Autodesk Inventor part; units mm, degrees
(part 9 of 12)
  line L7174 (-19.2358, 25.9762) -> (-19.2358, 24.9762)
  line L7175 (-19.8581, 24.9762) -> (-20.8581, 24.9762)
  line L7176 (-20.8581, 24.9762) -> (-20.8581, 25.9762)
  line L7177 (-20.8581, 25.9762) -> (-19.8581, 25.9762)
  line L7178 (-19.8581, 25.9762) -> (-19.8581, 24.9762)
  line L7179 (-20.4804, 24.9762) -> (-21.4804, 24.9762)
  line L7180 (-21.4804, 24.9762) -> (-21.4804, 25.9762)
  line L7181 (-21.4804, 25.9762) -> (-20.4804, 25.9762)
  line L7182 (-20.4804, 25.9762) -> (-20.4804, 24.9762)
  line L7183 (-21.4837, 24.9762) -> (-22.4837, 24.9762)
  line L7184 (-22.4837, 24.9762) -> (-22.4837, 25.9762)
  line L7185 (-22.4837, 25.9762) -> (-21.4837, 25.9762)
  line L7186 (-21.4837, 25.9762) -> (-21.4837, 24.9762)
  line L7187 (-12.9239, 25.0016) -> (-13.9239, 25.0016)
  line L7188 (-13.9239, 25.0016) -> (-13.9239, 26.0016)
  line L7189 (-13.9239, 26.0016) -> (-12.9239, 26.0016)
  line L7190 (-12.9239, 26.0016) -> (-12.9239, 25.0016)
  line L7191 (-13.6478, 25.0016) -> (-14.6478, 25.0016)
  line L7192 (-14.6478, 25.0016) -> (-14.6478, 26.0016)
  line L7193 (-14.6478, 26.0016) -> (-13.6478, 26.0016)
  line L7194 (-13.6478, 26.0016) -> (-13.6478, 25.0016)
  line L7195 (-14.5622, 25.0016) -> (-15.5622, 25.0016)
  line L7196 (-15.5622, 25.0016) -> (-15.5622, 26.0016)
  line L7197 (-15.5622, 26.0016) -> (-14.5622, 26.0016)
  line L7198 (-14.5622, 26.0016) -> (-14.5622, 25.0016)
  line L7199 (-15.8449, 25.0016) -> (-16.8449, 25.0016)
  line L7200 (-16.8449, 25.0016) -> (-16.8449, 26.0016)
  line L7201 (-16.8449, 26.0016) -> (-15.8449, 26.0016)
  line L7202 (-15.8449, 26.0016) -> (-15.8449, 25.0016)
  line L7203 (-16.8228, 25.0016) -> (-17.8228, 25.0016)
  line L7204 (-17.8228, 25.0016) -> (-17.8228, 26.0016)
  line L7205 (-17.8228, 26.0016) -> (-16.8228, 26.0016)
  line L7206 (-16.8228, 26.0016) -> (-16.8228, 25.0016)
  line L7207 (-17.4324, 25.0016) -> (-18.4324, 25.0016)
  line L7208 (-18.4324, 25.0016) -> (-18.4324, 26.0016)
  line L7209 (-18.4324, 26.0016) -> (-17.4324, 26.0016)
  line L7210 (-17.4324, 26.0016) -> (-17.4324, 25.0016)
  line L7211 (-17.9404, 25.0016) -> (-18.9404, 25.0016)
  line L7212 (-18.9404, 25.0016) -> (-18.9404, 26.0016)
  line L7213 (-18.9404, 26.0016) -> (-17.9404, 26.0016)
  line L7214 (-17.9404, 26.0016) -> (-17.9404, 25.0016)
  line L7215 (-18.677, 25.0016) -> (-19.677, 25.0016)
  line L7216 (-19.677, 25.0016) -> (-19.677, 26.0016)
  line L7217 (-19.677, 26.0016) -> (-18.677, 26.0016)
  line L7218 (-18.677, 26.0016) -> (-18.677, 25.0016)
  line L7219 (-19.2485, 25.0016) -> (-20.2485, 25.0016)
  line L7220 (-20.2485, 25.0016) -> (-20.2485, 26.0016)
  line L7221 (-20.2485, 26.0016) -> (-19.2485, 26.0016)
  line L7222 (-19.2485, 26.0016) -> (-19.2485, 25.0016)
  line L7223 (-19.8454, 25.0016) -> (-20.8454, 25.0016)
  line L7224 (-20.8454, 25.0016) -> (-20.8454, 26.0016)
  line L7225 (-20.8454, 26.0016) -> (-19.8454, 26.0016)
  line L7226 (-19.8454, 26.0016) -> (-19.8454, 25.0016)
  line L7227 (-20.4804, 25.0016) -> (-21.4804, 25.0016)
  line L7228 (-21.4804, 25.0016) -> (-21.4804, 26.0016)
  line L7229 (-21.4804, 26.0016) -> (-20.4804, 26.0016)
  line L7230 (-20.4804, 26.0016) -> (-20.4804, 25.0016)
  line L7231 (-21.4837, 25.0016) -> (-22.4837, 25.0016)
  line L7232 (-22.4837, 25.0016) -> (-22.4837, 26.0016)
  line L7233 (-22.4837, 26.0016) -> (-21.4837, 26.0016)
  line L7234 (-21.4837, 26.0016) -> (-21.4837, 25.0016)
  line L7235 (-12.9239, 25.027) -> (-13.9239, 25.027)
  line L7236 (-13.9239, 25.027) -> (-13.9239, 26.027)
  line L7237 (-13.9239, 26.027) -> (-12.9239, 26.027)
  line L7238 (-12.9239, 26.027) -> (-12.9239, 25.027)
  line L7239 (-13.6224, 25.027) -> (-14.6224, 25.027)
  line L7240 (-14.6224, 25.027) -> (-14.6224, 26.027)
  line L7241 (-14.6224, 26.027) -> (-13.6224, 26.027)
  line L7242 (-13.6224, 26.027) -> (-13.6224, 25.027)
  line L7243 (-14.5495, 25.027) -> (-15.5495, 25.027)
  line L7244 (-15.5495, 25.027) -> (-15.5495, 26.027)
  line L7245 (-15.5495, 26.027) -> (-14.5495, 26.027)
  line L7246 (-14.5495, 26.027) -> (-14.5495, 25.027)
  line L7247 (-15.5528, 25.027) -> (-16.5528, 25.027)
  line L7248 (-16.5528, 25.027) -> (-16.5528, 26.027)
  line L7249 (-16.5528, 26.027) -> (-15.5528, 26.027)
  line L7250 (-15.5528, 26.027) -> (-15.5528, 25.027)
  line L7251 (-16.1751, 25.027) -> (-17.1751, 25.027)
  line L7252 (-17.1751, 25.027) -> (-17.1751, 26.027)
  line L7253 (-17.1751, 26.027) -> (-16.1751, 26.027)
  line L7254 (-16.1751, 26.027) -> (-16.1751, 25.027)
  line L7255 (-16.7974, 25.027) -> (-17.7974, 25.027)
  line L7256 (-17.7974, 25.027) -> (-17.7974, 26.027)
  line L7257 (-17.7974, 26.027) -> (-16.7974, 26.027)
  line L7258 (-16.7974, 26.027) -> (-16.7974, 25.027)
  line L7259 (-17.4832, 25.027) -> (-18.4832, 25.027)
  line L7260 (-18.4832, 25.027) -> (-18.4832, 26.027)
  line L7261 (-18.4832, 26.027) -> (-17.4832, 26.027)
  line L7262 (-17.4832, 26.027) -> (-17.4832, 25.027)
  line L7263 (-17.9404, 25.027) -> (-18.9404, 25.027)
  line L7264 (-18.9404, 25.027) -> (-18.9404, 26.027)
  line L7265 (-18.9404, 26.027) -> (-17.9404, 26.027)
  line L7266 (-17.9404, 26.027) -> (-17.9404, 25.027)
  line L7267 (-18.677, 25.027) -> (-19.677, 25.027)
  line L7268 (-19.677, 25.027) -> (-19.677, 26.027)
  line L7269 (-19.677, 26.027) -> (-18.677, 26.027)
  line L7270 (-18.677, 26.027) -> (-18.677, 25.027)
  line L7271 (-19.2485, 25.027) -> (-20.2485, 25.027)
  line L7272 (-20.2485, 25.027) -> (-20.2485, 26.027)
  line L7273 (-20.2485, 26.027) -> (-19.2485, 26.027)
  line L7274 (-19.2485, 26.027) -> (-19.2485, 25.027)
  line L7275 (-19.8581, 25.027) -> (-20.8581, 25.027)
  line L7276 (-20.8581, 25.027) -> (-20.8581, 26.027)
  line L7277 (-20.8581, 26.027) -> (-19.8581, 26.027)
  line L7278 (-19.8581, 26.027) -> (-19.8581, 25.027)
  line L7279 (-20.4804, 25.027) -> (-21.4804, 25.027)
  line L7280 (-21.4804, 25.027) -> (-21.4804, 26.027)
  line L7281 (-21.4804, 26.027) -> (-20.4804, 26.027)
  line L7282 (-20.4804, 26.027) -> (-20.4804, 25.027)
  line L7283 (-21.4964, 25.027) -> (-22.4964, 25.027)
  line L7284 (-22.4964, 25.027) -> (-22.4964, 26.027)
  line L7285 (-22.4964, 26.027) -> (-21.4964, 26.027)
  line L7286 (-21.4964, 26.027) -> (-21.4964, 25.027)
  line L7287 (-12.9112, 25.0524) -> (-13.9112, 25.0524)
  line L7288 (-13.9112, 25.0524) -> (-13.9112, 26.0524)
  line L7289 (-13.9112, 26.0524) -> (-12.9112, 26.0524)
  line L7290 (-12.9112, 26.0524) -> (-12.9112, 25.0524)
  line L7291 (-13.597, 25.0524) -> (-14.597, 25.0524)
  line L7292 (-14.597, 25.0524) -> (-14.597, 26.0524)
  line L7293 (-14.597, 26.0524) -> (-13.597, 26.0524)
  line L7294 (-13.597, 26.0524) -> (-13.597, 25.0524)
  line L7295 (-14.5241, 25.0524) -> (-15.5241, 25.0524)
  line L7296 (-15.5241, 25.0524) -> (-15.5241, 26.0524)
  line L7297 (-15.5241, 26.0524) -> (-14.5241, 26.0524)
  line L7298 (-14.5241, 26.0524) -> (-14.5241, 25.0524)
  line L7299 (-15.5274, 25.0524) -> (-16.5274, 25.0524)
  line L7300 (-16.5274, 25.0524) -> (-16.5274, 26.0524)
  line L7301 (-16.5274, 26.0524) -> (-15.5274, 26.0524)
  line L7302 (-15.5274, 26.0524) -> (-15.5274, 25.0524)
  line L7303 (-16.2005, 25.0524) -> (-17.2005, 25.0524)
  line L7304 (-17.2005, 25.0524) -> (-17.2005, 26.0524)
  line L7305 (-17.2005, 26.0524) -> (-16.2005, 26.0524)
  line L7306 (-16.2005, 26.0524) -> (-16.2005, 25.0524)
  line L7307 (-16.772, 25.0524) -> (-17.772, 25.0524)
  line L7308 (-17.772, 25.0524) -> (-17.772, 26.0524)
  line L7309 (-17.772, 26.0524) -> (-16.772, 26.0524)
  line L7310 (-16.772, 26.0524) -> (-16.772, 25.0524)
  line L7311 (-17.9404, 25.0524) -> (-18.9404, 25.0524)
  line L7312 (-18.9404, 25.0524) -> (-18.9404, 26.0524)
  line L7313 (-18.9404, 26.0524) -> (-17.9404, 26.0524)
  line L7314 (-17.9404, 26.0524) -> (-17.9404, 25.0524)
  line L7315 (-18.677, 25.0524) -> (-19.677, 25.0524)
  line L7316 (-19.677, 25.0524) -> (-19.677, 26.0524)
  line L7317 (-19.677, 26.0524) -> (-18.677, 26.0524)
  line L7318 (-18.677, 26.0524) -> (-18.677, 25.0524)
  line L7319 (-19.2485, 25.0524) -> (-20.2485, 25.0524)
  line L7320 (-20.2485, 25.0524) -> (-20.2485, 26.0524)
  line L7321 (-20.2485, 26.0524) -> (-19.2485, 26.0524)
  line L7322 (-19.2485, 26.0524) -> (-19.2485, 25.0524)
  line L7323 (-19.8581, 25.0524) -> (-20.8581, 25.0524)
  line L7324 (-20.8581, 25.0524) -> (-20.8581, 26.0524)
  line L7325 (-20.8581, 26.0524) -> (-19.8581, 26.0524)
  line L7326 (-19.8581, 26.0524) -> (-19.8581, 25.0524)
  line L7327 (-20.4804, 25.0524) -> (-21.4804, 25.0524)
  line L7328 (-21.4804, 25.0524) -> (-21.4804, 26.0524)
  line L7329 (-21.4804, 26.0524) -> (-20.4804, 26.0524)
  line L7330 (-20.4804, 26.0524) -> (-20.4804, 25.0524)
  line L7331 (-21.4837, 25.0524) -> (-22.4837, 25.0524)
  line L7332 (-22.4837, 25.0524) -> (-22.4837, 26.0524)
  line L7333 (-22.4837, 26.0524) -> (-21.4837, 26.0524)
  line L7334 (-21.4837, 26.0524) -> (-21.4837, 25.0524)
  line L7335 (-12.9112, 25.0778) -> (-13.9112, 25.0778)
  line L7336 (-13.9112, 25.0778) -> (-13.9112, 26.0778)
  line L7337 (-13.9112, 26.0778) -> (-12.9112, 26.0778)
  line L7338 (-12.9112, 26.0778) -> (-12.9112, 25.0778)
  line L7339 (-13.5843, 25.0778) -> (-14.5843, 25.0778)
  line L7340 (-14.5843, 25.0778) -> (-14.5843, 26.0778)
  line L7341 (-14.5843, 26.0778) -> (-13.5843, 26.0778)
  line L7342 (-13.5843, 26.0778) -> (-13.5843, 25.0778)
  line L7343 (-14.5241, 25.0778) -> (-15.5241, 25.0778)
  line L7344 (-15.5241, 25.0778) -> (-15.5241, 26.0778)
  line L7345 (-15.5241, 26.0778) -> (-14.5241, 26.0778)
  line L7346 (-14.5241, 26.0778) -> (-14.5241, 25.0778)
  line L7347 (-15.5147, 25.0778) -> (-16.5147, 25.0778)
  line L7348 (-16.5147, 25.0778) -> (-16.5147, 26.0778)
  line L7349 (-16.5147, 26.0778) -> (-15.5147, 26.0778)
  line L7350 (-15.5147, 26.0778) -> (-15.5147, 25.0778)
  line L7351 (-16.2005, 25.0778) -> (-17.2005, 25.0778)
  line L7352 (-17.2005, 25.0778) -> (-17.2005, 26.0778)
  line L7353 (-17.2005, 26.0778) -> (-16.2005, 26.0778)
  line L7354 (-16.2005, 26.0778) -> (-16.2005, 25.0778)
  line L7355 (-16.7466, 25.0778) -> (-17.7466, 25.0778)
  line L7356 (-17.7466, 25.0778) -> (-17.7466, 26.0778)
  line L7357 (-17.7466, 26.0778) -> (-16.7466, 26.0778)
  line L7358 (-16.7466, 26.0778) -> (-16.7466, 25.0778)
  line L7359 (-17.9404, 25.0778) -> (-18.9404, 25.0778)
  line L7360 (-18.9404, 25.0778) -> (-18.9404, 26.0778)
  line L7361 (-18.9404, 26.0778) -> (-17.9404, 26.0778)
  line L7362 (-17.9404, 26.0778) -> (-17.9404, 25.0778)
  line L7363 (-18.677, 25.0778) -> (-19.677, 25.0778)
  line L7364 (-19.677, 25.0778) -> (-19.677, 26.0778)
  line L7365 (-19.677, 26.0778) -> (-18.677, 26.0778)
  line L7366 (-18.677, 26.0778) -> (-18.677, 25.0778)
  line L7367 (-19.2485, 25.0778) -> (-20.2485, 25.0778)
  line L7368 (-20.2485, 25.0778) -> (-20.2485, 26.0778)
  line L7369 (-20.2485, 26.0778) -> (-19.2485, 26.0778)
  line L7370 (-19.2485, 26.0778) -> (-19.2485, 25.0778)
  line L7371 (-19.8581, 25.0778) -> (-20.8581, 25.0778)
  line L7372 (-20.8581, 25.0778) -> (-20.8581, 26.0778)
  line L7373 (-20.8581, 26.0778) -> (-19.8581, 26.0778)
  line L7374 (-19.8581, 26.0778) -> (-19.8581, 25.0778)
  line L7375 (-20.4804, 25.0778) -> (-21.4804, 25.0778)
  line L7376 (-21.4804, 25.0778) -> (-21.4804, 26.0778)
  line L7377 (-21.4804, 26.0778) -> (-20.4804, 26.0778)
  line L7378 (-20.4804, 26.0778) -> (-20.4804, 25.0778)
  line L7379 (-21.4964, 25.0778) -> (-22.4964, 25.0778)
  line L7380 (-22.4964, 25.0778) -> (-22.4964, 26.0778)
  line L7381 (-22.4964, 26.0778) -> (-21.4964, 26.0778)
  line L7382 (-21.4964, 26.0778) -> (-21.4964, 25.0778)
  line L7383 (-12.8985, 25.1032) -> (-13.8985, 25.1032)
  line L7384 (-13.8985, 25.1032) -> (-13.8985, 26.1032)
  line L7385 (-13.8985, 26.1032) -> (-12.8985, 26.1032)
  line L7386 (-12.8985, 26.1032) -> (-12.8985, 25.1032)
  line L7387 (-13.5589, 25.1032) -> (-14.5589, 25.1032)
  line L7388 (-14.5589, 25.1032) -> (-14.5589, 26.1032)
  line L7389 (-14.5589, 26.1032) -> (-13.5589, 26.1032)
  line L7390 (-13.5589, 26.1032) -> (-13.5589, 25.1032)
  line L7391 (-14.4987, 25.1032) -> (-15.4987, 25.1032)
  line L7392 (-15.4987, 25.1032) -> (-15.4987, 26.1032)
  line L7393 (-15.4987, 26.1032) -> (-14.4987, 26.1032)
  line L7394 (-14.4987, 26.1032) -> (-14.4987, 25.1032)
  line L7395 (-15.5147, 25.1032) -> (-16.5147, 25.1032)
  line L7396 (-16.5147, 25.1032) -> (-16.5147, 26.1032)
  line L7397 (-16.5147, 26.1032) -> (-15.5147, 26.1032)
  line L7398 (-15.5147, 26.1032) -> (-15.5147, 25.1032)
  line L7399 (-16.2132, 25.1032) -> (-17.2132, 25.1032)
  line L7400 (-17.2132, 25.1032) -> (-17.2132, 26.1032)
  line L7401 (-17.2132, 26.1032) -> (-16.2132, 26.1032)
  line L7402 (-16.2132, 26.1032) -> (-16.2132, 25.1032)
  line L7403 (-16.7466, 25.1032) -> (-17.7466, 25.1032)
  line L7404 (-17.7466, 25.1032) -> (-17.7466, 26.1032)
  line L7405 (-17.7466, 26.1032) -> (-16.7466, 26.1032)
  line L7406 (-16.7466, 26.1032) -> (-16.7466, 25.1032)
  line L7407 (-17.9404, 25.1032) -> (-18.9404, 25.1032)
  line L7408 (-18.9404, 25.1032) -> (-18.9404, 26.1032)
  line L7409 (-18.9404, 26.1032) -> (-17.9404, 26.1032)
  line L7410 (-17.9404, 26.1032) -> (-17.9404, 25.1032)
  line L7411 (-18.677, 25.1032) -> (-19.677, 25.1032)
  line L7412 (-19.677, 25.1032) -> (-19.677, 26.1032)
  line L7413 (-19.677, 26.1032) -> (-18.677, 26.1032)
  line L7414 (-18.677, 26.1032) -> (-18.677, 25.1032)
  line L7415 (-19.2485, 25.1032) -> (-20.2485, 25.1032)
  line L7416 (-20.2485, 25.1032) -> (-20.2485, 26.1032)
  line L7417 (-20.2485, 26.1032) -> (-19.2485, 26.1032)
  line L7418 (-19.2485, 26.1032) -> (-19.2485, 25.1032)
  line L7419 (-19.8581, 25.1032) -> (-20.8581, 25.1032)
  line L7420 (-20.8581, 25.1032) -> (-20.8581, 26.1032)
  line L7421 (-20.8581, 26.1032) -> (-19.8581, 26.1032)
  line L7422 (-19.8581, 26.1032) -> (-19.8581, 25.1032)
  line L7423 (-20.4804, 25.1032) -> (-21.4804, 25.1032)
  line L7424 (-21.4804, 25.1032) -> (-21.4804, 26.1032)
  line L7425 (-21.4804, 26.1032) -> (-20.4804, 26.1032)
  line L7426 (-20.4804, 26.1032) -> (-20.4804, 25.1032)
  line L7427 (-21.3059, 25.1032) -> (-22.3059, 25.1032)
  line L7428 (-22.3059, 25.1032) -> (-22.3059, 26.1032)
  line L7429 (-22.3059, 26.1032) -> (-21.3059, 26.1032)
  line L7430 (-21.3059, 26.1032) -> (-21.3059, 25.1032)
  line L7431 (-21.6869, 25.1032) -> (-22.6869, 25.1032)
  line L7432 (-22.6869, 25.1032) -> (-22.6869, 26.1032)
  line L7433 (-22.6869, 26.1032) -> (-21.6869, 26.1032)
  line L7434 (-21.6869, 26.1032) -> (-21.6869, 25.1032)
  line L7435 (-12.8985, 25.1286) -> (-13.8985, 25.1286)
  line L7436 (-13.8985, 25.1286) -> (-13.8985, 26.1286)
  line L7437 (-13.8985, 26.1286) -> (-12.8985, 26.1286)
  line L7438 (-12.8985, 26.1286) -> (-12.8985, 25.1286)
  line L7439 (-13.5335, 25.1286) -> (-14.5335, 25.1286)
  line L7440 (-14.5335, 25.1286) -> (-14.5335, 26.1286)
  line L7441 (-14.5335, 26.1286) -> (-13.5335, 26.1286)
  line L7442 (-13.5335, 26.1286) -> (-13.5335, 25.1286)
  line L7443 (-14.486, 25.1286) -> (-15.486, 25.1286)
  line L7444 (-15.486, 25.1286) -> (-15.486, 26.1286)
  line L7445 (-15.486, 26.1286) -> (-14.486, 26.1286)
  line L7446 (-14.486, 26.1286) -> (-14.486, 25.1286)
  line L7447 (-15.502, 25.1286) -> (-16.502, 25.1286)
  line L7448 (-16.502, 25.1286) -> (-16.502, 26.1286)
  line L7449 (-16.502, 26.1286) -> (-15.502, 26.1286)
  line L7450 (-15.502, 26.1286) -> (-15.502, 25.1286)
  line L7451 (-16.2386, 25.1286) -> (-17.2386, 25.1286)
  line L7452 (-17.2386, 25.1286) -> (-17.2386, 26.1286)
  line L7453 (-17.2386, 26.1286) -> (-16.2386, 26.1286)
  line L7454 (-16.2386, 26.1286) -> (-16.2386, 25.1286)
  line L7455 (-16.7466, 25.1286) -> (-17.7466, 25.1286)
  line L7456 (-17.7466, 25.1286) -> (-17.7466, 26.1286)
  line L7457 (-17.7466, 26.1286) -> (-16.7466, 26.1286)
  line L7458 (-16.7466, 26.1286) -> (-16.7466, 25.1286)
  line L7459 (-17.9404, 25.1286) -> (-18.9404, 25.1286)
  line L7460 (-18.9404, 25.1286) -> (-18.9404, 26.1286)
  line L7461 (-18.9404, 26.1286) -> (-17.9404, 26.1286)
  line L7462 (-17.9404, 26.1286) -> (-17.9404, 25.1286)
  line L7463 (-18.677, 25.1286) -> (-19.677, 25.1286)
  line L7464 (-19.677, 25.1286) -> (-19.677, 26.1286)
  line L7465 (-19.677, 26.1286) -> (-18.677, 26.1286)
  line L7466 (-18.677, 26.1286) -> (-18.677, 25.1286)
  line L7467 (-19.2485, 25.1286) -> (-20.2485, 25.1286)
  line L7468 (-20.2485, 25.1286) -> (-20.2485, 26.1286)
  line L7469 (-20.2485, 26.1286) -> (-19.2485, 26.1286)
  line L7470 (-19.2485, 26.1286) -> (-19.2485, 25.1286)
  line L7471 (-19.8581, 25.1286) -> (-20.8581, 25.1286)
  line L7472 (-20.8581, 25.1286) -> (-20.8581, 26.1286)
  line L7473 (-20.8581, 26.1286) -> (-19.8581, 26.1286)
  line L7474 (-19.8581, 26.1286) -> (-19.8581, 25.1286)
  line L7475 (-20.4804, 25.1286) -> (-21.4804, 25.1286)
  line L7476 (-21.4804, 25.1286) -> (-21.4804, 26.1286)
  line L7477 (-21.4804, 26.1286) -> (-20.4804, 26.1286)
  line L7478 (-20.4804, 26.1286) -> (-20.4804, 25.1286)
  line L7479 (-21.2932, 25.1286) -> (-22.2932, 25.1286)
  line L7480 (-22.2932, 25.1286) -> (-22.2932, 26.1286)
  line L7481 (-22.2932, 26.1286) -> (-21.2932, 26.1286)
  line L7482 (-21.2932, 26.1286) -> (-21.2932, 25.1286)
  line L7483 (-21.6996, 25.1286) -> (-22.6996, 25.1286)
  line L7484 (-22.6996, 25.1286) -> (-22.6996, 26.1286)
  line L7485 (-22.6996, 26.1286) -> (-21.6996, 26.1286)
  line L7486 (-21.6996, 26.1286) -> (-21.6996, 25.1286)
  line L7487 (-12.8858, 25.154) -> (-13.8858, 25.154)
  line L7488 (-13.8858, 25.154) -> (-13.8858, 26.154)
  line L7489 (-13.8858, 26.154) -> (-12.8858, 26.154)
  line L7490 (-12.8858, 26.154) -> (-12.8858, 25.154)
  line L7491 (-13.5208, 25.154) -> (-14.5208, 25.154)
  line L7492 (-14.5208, 25.154) -> (-14.5208, 26.154)
  line L7493 (-14.5208, 26.154) -> (-13.5208, 26.154)
  line L7494 (-13.5208, 26.154) -> (-13.5208, 25.154)
  line L7495 (-14.4606, 25.154) -> (-15.4606, 25.154)
  line L7496 (-15.4606, 25.154) -> (-15.4606, 26.154)
  line L7497 (-15.4606, 26.154) -> (-14.4606, 26.154)
  line L7498 (-14.4606, 26.154) -> (-14.4606, 25.154)
  line L7499 (-15.502, 25.154) -> (-16.502, 25.154)
  line L7500 (-16.502, 25.154) -> (-16.502, 26.154)
  line L7501 (-16.502, 26.154) -> (-15.502, 26.154)
  line L7502 (-15.502, 26.154) -> (-15.502, 25.154)
  line L7503 (-16.2386, 25.154) -> (-17.2386, 25.154)
  line L7504 (-17.2386, 25.154) -> (-17.2386, 26.154)
  line L7505 (-17.2386, 26.154) -> (-16.2386, 26.154)
  line L7506 (-16.2386, 26.154) -> (-16.2386, 25.154)
  line L7507 (-16.7339, 25.154) -> (-17.7339, 25.154)
  line L7508 (-17.7339, 25.154) -> (-17.7339, 26.154)
  line L7509 (-17.7339, 26.154) -> (-16.7339, 26.154)
  line L7510 (-16.7339, 26.154) -> (-16.7339, 25.154)
  line L7511 (-17.9531, 25.154) -> (-18.9531, 25.154)
  line L7512 (-18.9531, 25.154) -> (-18.9531, 26.154)
  line L7513 (-18.9531, 26.154) -> (-17.9531, 26.154)
  line L7514 (-17.9531, 26.154) -> (-17.9531, 25.154)
  line L7515 (-18.677, 25.154) -> (-19.677, 25.154)
  line L7516 (-19.677, 25.154) -> (-19.677, 26.154)
  line L7517 (-19.677, 26.154) -> (-18.677, 26.154)
  line L7518 (-18.677, 26.154) -> (-18.677, 25.154)
  line L7519 (-19.2485, 25.154) -> (-20.2485, 25.154)
  line L7520 (-20.2485, 25.154) -> (-20.2485, 26.154)
  line L7521 (-20.2485, 26.154) -> (-19.2485, 26.154)
  line L7522 (-19.2485, 26.154) -> (-19.2485, 25.154)
  line L7523 (-19.8581, 25.154) -> (-20.8581, 25.154)
  line L7524 (-20.8581, 25.154) -> (-20.8581, 26.154)
  line L7525 (-20.8581, 26.154) -> (-19.8581, 26.154)
  line L7526 (-19.8581, 26.154) -> (-19.8581, 25.154)
  line L7527 (-20.4804, 25.154) -> (-21.4804, 25.154)
  line L7528 (-21.4804, 25.154) -> (-21.4804, 26.154)
  line L7529 (-21.4804, 26.154) -> (-20.4804, 26.154)
  line L7530 (-20.4804, 26.154) -> (-20.4804, 25.154)
  line L7531 (-21.2932, 25.154) -> (-22.2932, 25.154)
  line L7532 (-22.2932, 25.154) -> (-22.2932, 26.154)
  line L7533 (-22.2932, 26.154) -> (-21.2932, 26.154)
  line L7534 (-21.2932, 26.154) -> (-21.2932, 25.154)
  line L7535 (-21.7123, 25.154) -> (-22.7123, 25.154)
  line L7536 (-22.7123, 25.154) -> (-22.7123, 26.154)
  line L7537 (-22.7123, 26.154) -> (-21.7123, 26.154)
  line L7538 (-21.7123, 26.154) -> (-21.7123, 25.154)
  line L7539 (-12.8858, 25.1794) -> (-13.8858, 25.1794)
  line L7540 (-13.8858, 25.1794) -> (-13.8858, 26.1794)
  line L7541 (-13.8858, 26.1794) -> (-12.8858, 26.1794)
  line L7542 (-12.8858, 26.1794) -> (-12.8858, 25.1794)
  line L7543 (-13.4954, 25.1794) -> (-14.4954, 25.1794)
  line L7544 (-14.4954, 25.1794) -> (-14.4954, 26.1794)
  line L7545 (-14.4954, 26.1794) -> (-13.4954, 26.1794)
  line L7546 (-13.4954, 26.1794) -> (-13.4954, 25.1794)
  line L7547 (-14.4733, 25.1794) -> (-15.4733, 25.1794)
  line L7548 (-15.4733, 25.1794) -> (-15.4733, 26.1794)
  line L7549 (-15.4733, 26.1794) -> (-14.4733, 26.1794)
  line L7550 (-14.4733, 26.1794) -> (-14.4733, 25.1794)
  line L7551 (-15.502, 25.1794) -> (-16.502, 25.1794)
  line L7552 (-16.502, 25.1794) -> (-16.502, 26.1794)
  line L7553 (-16.502, 26.1794) -> (-15.502, 26.1794)
  line L7554 (-15.502, 26.1794) -> (-15.502, 25.1794)
  line L7555 (-16.2386, 25.1794) -> (-17.2386, 25.1794)
  line L7556 (-17.2386, 25.1794) -> (-17.2386, 26.1794)
  line L7557 (-17.2386, 26.1794) -> (-16.2386, 26.1794)
  line L7558 (-16.2386, 26.1794) -> (-16.2386, 25.1794)
  line L7559 (-16.7339, 25.1794) -> (-17.7339, 25.1794)
  line L7560 (-17.7339, 25.1794) -> (-17.7339, 26.1794)
  line L7561 (-17.7339, 26.1794) -> (-16.7339, 26.1794)
  line L7562 (-16.7339, 26.1794) -> (-16.7339, 25.1794)
  line L7563 (-17.9531, 25.1794) -> (-18.9531, 25.1794)
  line L7564 (-18.9531, 25.1794) -> (-18.9531, 26.1794)
  line L7565 (-18.9531, 26.1794) -> (-17.9531, 26.1794)
  line L7566 (-17.9531, 26.1794) -> (-17.9531, 25.1794)
  line L7567 (-18.677, 25.1794) -> (-19.677, 25.1794)
  line L7568 (-19.677, 25.1794) -> (-19.677, 26.1794)
  line L7569 (-19.677, 26.1794) -> (-18.677, 26.1794)
  line L7570 (-18.677, 26.1794) -> (-18.677, 25.1794)
  line L7571 (-19.2485, 25.1794) -> (-20.2485, 25.1794)
  line L7572 (-20.2485, 25.1794) -> (-20.2485, 26.1794)
  line L7573 (-20.2485, 26.1794) -> (-19.2485, 26.1794)
  line L7574 (-19.2485, 26.1794) -> (-19.2485, 25.1794)
  line L7575 (-19.8708, 25.1794) -> (-20.8708, 25.1794)
  line L7576 (-20.8708, 25.1794) -> (-20.8708, 26.1794)
  line L7577 (-20.8708, 26.1794) -> (-19.8708, 26.1794)
  line L7578 (-19.8708, 26.1794) -> (-19.8708, 25.1794)
  line L7579 (-20.4804, 25.1794) -> (-21.4804, 25.1794)
  line L7580 (-21.4804, 25.1794) -> (-21.4804, 26.1794)
  line L7581 (-21.4804, 26.1794) -> (-20.4804, 26.1794)
  line L7582 (-20.4804, 26.1794) -> (-20.4804, 25.1794)
  line L7583 (-21.2805, 25.1794) -> (-22.2805, 25.1794)
  line L7584 (-22.2805, 25.1794) -> (-22.2805, 26.1794)
  line L7585 (-22.2805, 26.1794) -> (-21.2805, 26.1794)
  line L7586 (-21.2805, 26.1794) -> (-21.2805, 25.1794)
  line L7587 (-21.725, 25.1794) -> (-22.725, 25.1794)
  line L7588 (-22.725, 25.1794) -> (-22.725, 26.1794)
  line L7589 (-22.725, 26.1794) -> (-21.725, 26.1794)
  line L7590 (-21.725, 26.1794) -> (-21.725, 25.1794)
  line L7591 (-12.8731, 25.2048) -> (-13.8731, 25.2048)
  line L7592 (-13.8731, 25.2048) -> (-13.8731, 26.2048)
  line L7593 (-13.8731, 26.2048) -> (-12.8731, 26.2048)
  line L7594 (-12.8731, 26.2048) -> (-12.8731, 25.2048)
  line L7595 (-13.47, 25.2048) -> (-14.47, 25.2048)
  line L7596 (-14.47, 25.2048) -> (-14.47, 26.2048)
  line L7597 (-14.47, 26.2048) -> (-13.47, 26.2048)
  line L7598 (-13.47, 26.2048) -> (-13.47, 25.2048)
  line L7599 (-14.4987, 25.2048) -> (-15.4987, 25.2048)
  line L7600 (-15.4987, 25.2048) -> (-15.4987, 26.2048)
  line L7601 (-15.4987, 26.2048) -> (-14.4987, 26.2048)
  line L7602 (-14.4987, 26.2048) -> (-14.4987, 25.2048)
  line L7603 (-15.502, 25.2048) -> (-16.502, 25.2048)
  line L7604 (-16.502, 25.2048) -> (-16.502, 26.2048)
  line L7605 (-16.502, 26.2048) -> (-15.502, 26.2048)
  line L7606 (-15.502, 26.2048) -> (-15.502, 25.2048)
  line L7607 (-16.2386, 25.2048) -> (-17.2386, 25.2048)
  line L7608 (-17.2386, 25.2048) -> (-17.2386, 26.2048)
  line L7609 (-17.2386, 26.2048) -> (-16.2386, 26.2048)
  line L7610 (-16.2386, 26.2048) -> (-16.2386, 25.2048)
  line L7611 (-16.7339, 25.2048) -> (-17.7339, 25.2048)
  line L7612 (-17.7339, 25.2048) -> (-17.7339, 26.2048)
  line L7613 (-17.7339, 26.2048) -> (-16.7339, 26.2048)
  line L7614 (-16.7339, 26.2048) -> (-16.7339, 25.2048)
  line L7615 (-17.9531, 25.2048) -> (-18.9531, 25.2048)
  line L7616 (-18.9531, 25.2048) -> (-18.9531, 26.2048)
  line L7617 (-18.9531, 26.2048) -> (-17.9531, 26.2048)
  line L7618 (-17.9531, 26.2048) -> (-17.9531, 25.2048)
  line L7619 (-18.677, 25.2048) -> (-19.677, 25.2048)
  line L7620 (-19.677, 25.2048) -> (-19.677, 26.2048)
  line L7621 (-19.677, 26.2048) -> (-18.677, 26.2048)
  line L7622 (-18.677, 26.2048) -> (-18.677, 25.2048)
  line L7623 (-19.2612, 25.2048) -> (-20.2612, 25.2048)
  line L7624 (-20.2612, 25.2048) -> (-20.2612, 26.2048)
  line L7625 (-20.2612, 26.2048) -> (-19.2612, 26.2048)
  line L7626 (-19.2612, 26.2048) -> (-19.2612, 25.2048)
  line L7627 (-19.8708, 25.2048) -> (-20.8708, 25.2048)
  line L7628 (-20.8708, 25.2048) -> (-20.8708, 26.2048)
  line L7629 (-20.8708, 26.2048) -> (-19.8708, 26.2048)
  line L7630 (-19.8708, 26.2048) -> (-19.8708, 25.2048)
  line L7631 (-20.4804, 25.2048) -> (-21.4804, 25.2048)
  line L7632 (-21.4804, 25.2048) -> (-21.4804, 26.2048)
  line L7633 (-21.4804, 26.2048) -> (-20.4804, 26.2048)
  line L7634 (-20.4804, 26.2048) -> (-20.4804, 25.2048)
  line L7635 (-21.2678, 25.2048) -> (-22.2678, 25.2048)
  line L7636 (-22.2678, 25.2048) -> (-22.2678, 26.2048)
  line L7637 (-22.2678, 26.2048) -> (-21.2678, 26.2048)
  line L7638 (-21.2678, 26.2048) -> (-21.2678, 25.2048)
  line L7639 (-21.725, 25.2048) -> (-22.725, 25.2048)
  line L7640 (-22.725, 25.2048) -> (-22.725, 26.2048)
  line L7641 (-22.725, 26.2048) -> (-21.725, 26.2048)
  line L7642 (-21.725, 26.2048) -> (-21.725, 25.2048)
  line L7643 (-12.8731, 25.2302) -> (-13.8731, 25.2302)
  line L7644 (-13.8731, 25.2302) -> (-13.8731, 26.2302)
  line L7645 (-13.8731, 26.2302) -> (-12.8731, 26.2302)
  line L7646 (-12.8731, 26.2302) -> (-12.8731, 25.2302)
  line L7647 (-13.9319, 25.7175) -> (-13.9573, 25.7175)
  line L7648 (-13.9573, 25.7175) -> (-13.9573, 25.7429)
  line L7649 (-13.9573, 25.7429) -> (-13.9319, 25.7429)
  line L7650 (-13.9319, 25.7429) -> (-13.9319, 25.7175)
  line L7651 (-14.5241, 25.2302) -> (-15.5241, 25.2302)
  line L7652 (-15.5241, 25.2302) -> (-15.5241, 26.2302)
  line L7653 (-15.5241, 26.2302) -> (-14.5241, 26.2302)
  line L7654 (-14.5241, 26.2302) -> (-14.5241, 25.2302)
  line L7655 (-15.4893, 25.2302) -> (-16.4893, 25.2302)
  line L7656 (-16.4893, 25.2302) -> (-16.4893, 26.2302)
  line L7657 (-16.4893, 26.2302) -> (-15.4893, 26.2302)
  line L7658 (-15.4893, 26.2302) -> (-15.4893, 25.2302)
  line L7659 (-16.2386, 25.2302) -> (-17.2386, 25.2302)
  line L7660 (-17.2386, 25.2302) -> (-17.2386, 26.2302)
  line L7661 (-17.2386, 26.2302) -> (-16.2386, 26.2302)
  line L7662 (-16.2386, 26.2302) -> (-16.2386, 25.2302)
  line L7663 (-17.0768, 25.2302) -> (-18.0768, 25.2302)
  line L7664 (-18.0768, 25.2302) -> (-18.0768, 26.2302)
  line L7665 (-18.0768, 26.2302) -> (-17.0768, 26.2302)
  line L7666 (-17.0768, 26.2302) -> (-17.0768, 25.2302)
  line L7667 (-17.9658, 25.2302) -> (-18.9658, 25.2302)
  line L7668 (-18.9658, 25.2302) -> (-18.9658, 26.2302)
  line L7669 (-18.9658, 26.2302) -> (-17.9658, 26.2302)
  line L7670 (-17.9658, 26.2302) -> (-17.9658, 25.2302)
  line L7671 (-18.6897, 25.2302) -> (-19.6897, 25.2302)
  line L7672 (-19.6897, 25.2302) -> (-19.6897, 26.2302)
  line L7673 (-19.6897, 26.2302) -> (-18.6897, 26.2302)
  line L7674 (-18.6897, 26.2302) -> (-18.6897, 25.2302)
  line L7675 (-19.2612, 25.2302) -> (-20.2612, 25.2302)
  line L7676 (-20.2612, 25.2302) -> (-20.2612, 26.2302)
  line L7677 (-20.2612, 26.2302) -> (-19.2612, 26.2302)
  line L7678 (-19.2612, 26.2302) -> (-19.2612, 25.2302)
  line L7679 (-19.8581, 25.2302) -> (-20.8581, 25.2302)
  line L7680 (-20.8581, 25.2302) -> (-20.8581, 26.2302)
  line L7681 (-20.8581, 26.2302) -> (-19.8581, 26.2302)
  line L7682 (-19.8581, 26.2302) -> (-19.8581, 25.2302)
  line L7683 (-20.4804, 25.2302) -> (-21.4804, 25.2302)
  line L7684 (-21.4804, 25.2302) -> (-21.4804, 26.2302)
  line L7685 (-21.4804, 26.2302) -> (-20.4804, 26.2302)
  line L7686 (-20.4804, 26.2302) -> (-20.4804, 25.2302)
  line L7687 (-21.2678, 25.2302) -> (-22.2678, 25.2302)
  line L7688 (-22.2678, 25.2302) -> (-22.2678, 26.2302)
  line L7689 (-22.2678, 26.2302) -> (-21.2678, 26.2302)
  line L7690 (-21.2678, 26.2302) -> (-21.2678, 25.2302)
  line L7691 (-21.7504, 25.2302) -> (-22.7504, 25.2302)
  line L7692 (-22.7504, 25.2302) -> (-22.7504, 26.2302)
  line L7693 (-22.7504, 26.2302) -> (-21.7504, 26.2302)
  line L7694 (-21.7504, 26.2302) -> (-21.7504, 25.2302)
  line L7695 (-12.8731, 25.2556) -> (-13.8731, 25.2556)
  line L7696 (-13.8731, 25.2556) -> (-13.8731, 26.2556)
  line L7697 (-13.8731, 26.2556) -> (-12.8731, 26.2556)
  line L7698 (-12.8731, 26.2556) -> (-12.8731, 25.2556)
  line L7699 (-14.5495, 25.2556) -> (-15.5495, 25.2556)
  line L7700 (-15.5495, 25.2556) -> (-15.5495, 26.2556)
  line L7701 (-15.5495, 26.2556) -> (-14.5495, 26.2556)
  line L7702 (-14.5495, 26.2556) -> (-14.5495, 25.2556)
  line L7703 (-15.4893, 25.2556) -> (-16.4893, 25.2556)
  line L7704 (-16.4893, 25.2556) -> (-16.4893, 26.2556)
  line L7705 (-16.4893, 26.2556) -> (-15.4893, 26.2556)
  line L7706 (-15.4893, 26.2556) -> (-15.4893, 25.2556)
  line L7707 (-16.2386, 25.2556) -> (-17.2386, 25.2556)
  line L7708 (-17.2386, 25.2556) -> (-17.2386, 26.2556)
  line L7709 (-17.2386, 26.2556) -> (-16.2386, 26.2556)
  line L7710 (-16.2386, 26.2556) -> (-16.2386, 25.2556)
  line L7711 (-17.0768, 25.2556) -> (-18.0768, 25.2556)
  line L7712 (-18.0768, 25.2556) -> (-18.0768, 26.2556)
  line L7713 (-18.0768, 26.2556) -> (-17.0768, 26.2556)
  line L7714 (-17.0768, 26.2556) -> (-17.0768, 25.2556)
  line L7715 (-17.9658, 25.2556) -> (-18.9658, 25.2556)
  line L7716 (-18.9658, 25.2556) -> (-18.9658, 26.2556)
  line L7717 (-18.9658, 26.2556) -> (-17.9658, 26.2556)
  line L7718 (-17.9658, 26.2556) -> (-17.9658, 25.2556)
  line L7719 (-18.6897, 25.2556) -> (-19.6897, 25.2556)
  line L7720 (-19.6897, 25.2556) -> (-19.6897, 26.2556)
  line L7721 (-19.6897, 26.2556) -> (-18.6897, 26.2556)
  line L7722 (-18.6897, 26.2556) -> (-18.6897, 25.2556)
  line L7723 (-19.2612, 25.2556) -> (-20.2612, 25.2556)
  line L7724 (-20.2612, 25.2556) -> (-20.2612, 26.2556)
  line L7725 (-20.2612, 26.2556) -> (-19.2612, 26.2556)
  line L7726 (-19.2612, 26.2556) -> (-19.2612, 25.2556)
  line L7727 (-19.8708, 25.2556) -> (-20.8708, 25.2556)
  line L7728 (-20.8708, 25.2556) -> (-20.8708, 26.2556)
  line L7729 (-20.8708, 26.2556) -> (-19.8708, 26.2556)
  line L7730 (-19.8708, 26.2556) -> (-19.8708, 25.2556)
  line L7731 (-20.4804, 25.2556) -> (-21.4804, 25.2556)
  line L7732 (-21.4804, 25.2556) -> (-21.4804, 26.2556)
  line L7733 (-21.4804, 26.2556) -> (-20.4804, 26.2556)
  line L7734 (-20.4804, 26.2556) -> (-20.4804, 25.2556)
  line L7735 (-21.2678, 25.2556) -> (-22.2678, 25.2556)
  line L7736 (-22.2678, 25.2556) -> (-22.2678, 26.2556)
  line L7737 (-22.2678, 26.2556) -> (-21.2678, 26.2556)
  line L7738 (-21.2678, 26.2556) -> (-21.2678, 25.2556)
  line L7739 (-21.7504, 25.2556) -> (-22.7504, 25.2556)
  line L7740 (-22.7504, 25.2556) -> (-22.7504, 26.2556)
  line L7741 (-22.7504, 26.2556) -> (-21.7504, 26.2556)
  line L7742 (-21.7504, 26.2556) -> (-21.7504, 25.2556)
  line L7743 (-12.8731, 25.281) -> (-13.8731, 25.281)
  line L7744 (-13.8731, 25.281) -> (-13.8731, 26.281)
  line L7745 (-13.8731, 26.281) -> (-12.8731, 26.281)
  line L7746 (-12.8731, 26.281) -> (-12.8731, 25.281)
  line L7747 (-14.5749, 25.281) -> (-15.5749, 25.281)
  line L7748 (-15.5749, 25.281) -> (-15.5749, 26.281)
  line L7749 (-15.5749, 26.281) -> (-14.5749, 26.281)
  line L7750 (-14.5749, 26.281) -> (-14.5749, 25.281)
  line L7751 (-15.4893, 25.281) -> (-16.4893, 25.281)
  line L7752 (-16.4893, 25.281) -> (-16.4893, 26.281)
  line L7753 (-16.4893, 26.281) -> (-15.4893, 26.281)
  line L7754 (-15.4893, 26.281) -> (-15.4893, 25.281)
  line L7755 (-16.2386, 25.281) -> (-17.2386, 25.281)
  line L7756 (-17.2386, 25.281) -> (-17.2386, 26.281)
  line L7757 (-17.2386, 26.281) -> (-16.2386, 26.281)
  line L7758 (-16.2386, 26.281) -> (-16.2386, 25.281)
  line L7759 (-17.0768, 25.281) -> (-18.0768, 25.281)
  line L7760 (-18.0768, 25.281) -> (-18.0768, 26.281)
  line L7761 (-18.0768, 26.281) -> (-17.0768, 26.281)
  line L7762 (-17.0768, 26.281) -> (-17.0768, 25.281)
  line L7763 (-17.9658, 25.281) -> (-18.9658, 25.281)
  line L7764 (-18.9658, 25.281) -> (-18.9658, 26.281)
  line L7765 (-18.9658, 26.281) -> (-17.9658, 26.281)
  line L7766 (-17.9658, 26.281) -> (-17.9658, 25.281)
  line L7767 (-18.6897, 25.281) -> (-19.6897, 25.281)
  line L7768 (-19.6897, 25.281) -> (-19.6897, 26.281)
  line L7769 (-19.6897, 26.281) -> (-18.6897, 26.281)
  line L7770 (-18.6897, 26.281) -> (-18.6897, 25.281)
  line L7771 (-19.2739, 25.281) -> (-20.2739, 25.281)
  line L7772 (-20.2739, 25.281) -> (-20.2739, 26.281)
  line L7773 (-20.2739, 26.281) -> (-19.2739, 26.281)
  line L7774 (-19.2739, 26.281) -> (-19.2739, 25.281)
  line L7775 (-19.8708, 25.281) -> (-20.8708, 25.281)
  line L7776 (-20.8708, 25.281) -> (-20.8708, 26.281)
  line L7777 (-20.8708, 26.281) -> (-19.8708, 26.281)
  line L7778 (-19.8708, 26.281) -> (-19.8708, 25.281)
  line L7779 (-20.4804, 25.281) -> (-21.4804, 25.281)
  line L7780 (-21.4804, 25.281) -> (-21.4804, 26.281)
  line L7781 (-21.4804, 26.281) -> (-20.4804, 26.281)
  line L7782 (-20.4804, 26.281) -> (-20.4804, 25.281)
  line L7783 (-21.2424, 25.281) -> (-22.2424, 25.281)
  line L7784 (-22.2424, 25.281) -> (-22.2424, 26.281)
  line L7785 (-22.2424, 26.281) -> (-21.2424, 26.281)
  line L7786 (-21.2424, 26.281) -> (-21.2424, 25.281)
  line L7787 (-21.7758, 25.281) -> (-22.7758, 25.281)
  line L7788 (-22.7758, 25.281) -> (-22.7758, 26.281)
  line L7789 (-22.7758, 26.281) -> (-21.7758, 26.281)
  line L7790 (-21.7758, 26.281) -> (-21.7758, 25.281)
  line L7791 (-12.8985, 25.3064) -> (-13.8985, 25.3064)
  line L7792 (-13.8985, 25.3064) -> (-13.8985, 26.3064)
  line L7793 (-13.8985, 26.3064) -> (-12.8985, 26.3064)
  line L7794 (-12.8985, 26.3064) -> (-12.8985, 25.3064)
  line L7795 (-14.6003, 25.3064) -> (-15.6003, 25.3064)
  line L7796 (-15.6003, 25.3064) -> (-15.6003, 26.3064)
  line L7797 (-15.6003, 26.3064) -> (-14.6003, 26.3064)
  line L7798 (-14.6003, 26.3064) -> (-14.6003, 25.3064)
  line L7799 (-15.502, 25.3064) -> (-16.502, 25.3064)
  line L7800 (-16.502, 25.3064) -> (-16.502, 26.3064)
  line L7801 (-16.502, 26.3064) -> (-15.502, 26.3064)
  line L7802 (-15.502, 26.3064) -> (-15.502, 25.3064)
  line L7803 (-16.2386, 25.3064) -> (-17.2386, 25.3064)
  line L7804 (-17.2386, 25.3064) -> (-17.2386, 26.3064)
  line L7805 (-17.2386, 26.3064) -> (-16.2386, 26.3064)
  line L7806 (-16.2386, 26.3064) -> (-16.2386, 25.3064)
  line L7807 (-17.0768, 25.3064) -> (-18.0768, 25.3064)
  line L7808 (-18.0768, 25.3064) -> (-18.0768, 26.3064)
  line L7809 (-18.0768, 26.3064) -> (-17.0768, 26.3064)
  line L7810 (-17.0768, 26.3064) -> (-17.0768, 25.3064)
  line L7811 (-17.9658, 25.3064) -> (-18.9658, 25.3064)
  line L7812 (-18.9658, 25.3064) -> (-18.9658, 26.3064)
  line L7813 (-18.9658, 26.3064) -> (-17.9658, 26.3064)
  line L7814 (-17.9658, 26.3064) -> (-17.9658, 25.3064)
  line L7815 (-18.677, 25.3064) -> (-19.677, 25.3064)
  line L7816 (-19.677, 25.3064) -> (-19.677, 26.3064)
  line L7817 (-19.677, 26.3064) -> (-18.677, 26.3064)
  line L7818 (-18.677, 26.3064) -> (-18.677, 25.3064)
  line L7819 (-19.2739, 25.3064) -> (-20.2739, 25.3064)
  line L7820 (-20.2739, 25.3064) -> (-20.2739, 26.3064)
  line L7821 (-20.2739, 26.3064) -> (-19.2739, 26.3064)
  line L7822 (-19.2739, 26.3064) -> (-19.2739, 25.3064)
  line L7823 (-19.7057, 25.3064) -> (-20.7057, 25.3064)
  line L7824 (-20.7057, 25.3064) -> (-20.7057, 26.3064)
  line L7825 (-20.7057, 26.3064) -> (-19.7057, 26.3064)
  line L7826 (-19.7057, 26.3064) -> (-19.7057, 25.3064)
  line L7827 (-20.0486, 25.3064) -> (-21.0486, 25.3064)
  line L7828 (-21.0486, 25.3064) -> (-21.0486, 26.3064)
  line L7829 (-21.0486, 26.3064) -> (-20.0486, 26.3064)
  line L7830 (-20.0486, 26.3064) -> (-20.0486, 25.3064)
  line L7831 (-20.4804, 25.3064) -> (-21.4804, 25.3064)
  line L7832 (-21.4804, 25.3064) -> (-21.4804, 26.3064)
  line L7833 (-21.4804, 26.3064) -> (-20.4804, 26.3064)
  line L7834 (-20.4804, 26.3064) -> (-20.4804, 25.3064)
  line L7835 (-21.2424, 25.3064) -> (-22.2424, 25.3064)
  line L7836 (-22.2424, 25.3064) -> (-22.2424, 26.3064)
  line L7837 (-22.2424, 26.3064) -> (-21.2424, 26.3064)
  line L7838 (-21.2424, 26.3064) -> (-21.2424, 25.3064)
  line L7839 (-21.7758, 25.3064) -> (-22.7758, 25.3064)
  line L7840 (-22.7758, 25.3064) -> (-22.7758, 26.3064)
  line L7841 (-22.7758, 26.3064) -> (-21.7758, 26.3064)
  line L7842 (-21.7758, 26.3064) -> (-21.7758, 25.3064)
  line L7843 (-12.9239, 25.3318) -> (-13.9239, 25.3318)
  line L7844 (-13.9239, 25.3318) -> (-13.9239, 26.3318)
  line L7845 (-13.9239, 26.3318) -> (-12.9239, 26.3318)
  line L7846 (-12.9239, 26.3318) -> (-12.9239, 25.3318)
  line L7847 (-14.6257, 25.3318) -> (-15.6257, 25.3318)
  line L7848 (-15.6257, 25.3318) -> (-15.6257, 26.3318)
  line L7849 (-15.6257, 26.3318) -> (-14.6257, 26.3318)
  line L7850 (-14.6257, 26.3318) -> (-14.6257, 25.3318)
  line L7851 (-15.502, 25.3318) -> (-16.502, 25.3318)
  line L7852 (-16.502, 25.3318) -> (-16.502, 26.3318)
  line L7853 (-16.502, 26.3318) -> (-15.502, 26.3318)
  line L7854 (-15.502, 26.3318) -> (-15.502, 25.3318)
  line L7855 (-16.2386, 25.3318) -> (-17.2386, 25.3318)
  line L7856 (-17.2386, 25.3318) -> (-17.2386, 26.3318)
  line L7857 (-17.2386, 26.3318) -> (-16.2386, 26.3318)
  line L7858 (-16.2386, 26.3318) -> (-16.2386, 25.3318)
  line L7859 (-17.0768, 25.3318) -> (-18.0768, 25.3318)
  line L7860 (-18.0768, 25.3318) -> (-18.0768, 26.3318)
  line L7861 (-18.0768, 26.3318) -> (-17.0768, 26.3318)
  line L7862 (-17.0768, 26.3318) -> (-17.0768, 25.3318)
  line L7863 (-17.9785, 25.3318) -> (-18.9785, 25.3318)
  line L7864 (-18.9785, 25.3318) -> (-18.9785, 26.3318)
  line L7865 (-18.9785, 26.3318) -> (-17.9785, 26.3318)
  line L7866 (-17.9785, 26.3318) -> (-17.9785, 25.3318)
  line L7867 (-18.6897, 25.3318) -> (-19.6897, 25.3318)
  line L7868 (-19.6897, 25.3318) -> (-19.6897, 26.3318)
  line L7869 (-19.6897, 26.3318) -> (-18.6897, 26.3318)
  line L7870 (-18.6897, 26.3318) -> (-18.6897, 25.3318)
  line L7871 (-19.2739, 25.3318) -> (-20.2739, 25.3318)
  line L7872 (-20.2739, 25.3318) -> (-20.2739, 26.3318)
  line L7873 (-20.2739, 26.3318) -> (-19.2739, 26.3318)
  line L7874 (-19.2739, 26.3318) -> (-19.2739, 25.3318)
  line L7875 (-19.693, 25.3318) -> (-20.693, 25.3318)
  line L7876 (-20.693, 25.3318) -> (-20.693, 26.3318)
  line L7877 (-20.693, 26.3318) -> (-19.693, 26.3318)
  line L7878 (-19.693, 26.3318) -> (-19.693, 25.3318)
  line L7879 (-20.0613, 25.3318) -> (-21.0613, 25.3318)
  line L7880 (-21.0613, 25.3318) -> (-21.0613, 26.3318)
  line L7881 (-21.0613, 26.3318) -> (-20.0613, 26.3318)
  line L7882 (-20.0613, 26.3318) -> (-20.0613, 25.3318)
  line L7883 (-20.4804, 25.3318) -> (-21.4804, 25.3318)
  line L7884 (-21.4804, 25.3318) -> (-21.4804, 26.3318)
  line L7885 (-21.4804, 26.3318) -> (-20.4804, 26.3318)
  line L7886 (-20.4804, 26.3318) -> (-20.4804, 25.3318)
  line L7887 (-21.2297, 25.3318) -> (-22.2297, 25.3318)
  line L7888 (-22.2297, 25.3318) -> (-22.2297, 26.3318)
  line L7889 (-22.2297, 26.3318) -> (-21.2297, 26.3318)
  line L7890 (-21.2297, 26.3318) -> (-21.2297, 25.3318)
  line L7891 (-21.8012, 25.3318) -> (-22.8012, 25.3318)
  line L7892 (-22.8012, 25.3318) -> (-22.8012, 26.3318)
  line L7893 (-22.8012, 26.3318) -> (-21.8012, 26.3318)
  line L7894 (-21.8012, 26.3318) -> (-21.8012, 25.3318)
  line L7895 (-12.9366, 25.3572) -> (-13.9366, 25.3572)
  line L7896 (-13.9366, 25.3572) -> (-13.9366, 26.3572)
  line L7897 (-13.9366, 26.3572) -> (-12.9366, 26.3572)
  line L7898 (-12.9366, 26.3572) -> (-12.9366, 25.3572)
  line L7899 (-14.6511, 25.3572) -> (-15.6511, 25.3572)
  line L7900 (-15.6511, 25.3572) -> (-15.6511, 26.3572)
  line L7901 (-15.6511, 26.3572) -> (-14.6511, 26.3572)
  line L7902 (-14.6511, 26.3572) -> (-14.6511, 25.3572)
  line L7903 (-15.502, 25.3572) -> (-16.502, 25.3572)
  line L7904 (-16.502, 25.3572) -> (-16.502, 26.3572)
  line L7905 (-16.502, 26.3572) -> (-15.502, 26.3572)
  line L7906 (-15.502, 26.3572) -> (-15.502, 25.3572)
  line L7907 (-16.2386, 25.3572) -> (-17.2386, 25.3572)
  line L7908 (-17.2386, 25.3572) -> (-17.2386, 26.3572)
  line L7909 (-17.2386, 26.3572) -> (-16.2386, 26.3572)
  line L7910 (-16.2386, 26.3572) -> (-16.2386, 25.3572)
  line L7911 (-16.7466, 25.3572) -> (-17.7466, 25.3572)
  line L7912 (-17.7466, 25.3572) -> (-17.7466, 26.3572)
  line L7913 (-17.7466, 26.3572) -> (-16.7466, 26.3572)
  line L7914 (-16.7466, 26.3572) -> (-16.7466, 25.3572)
  line L7915 (-17.4197, 25.3572) -> (-18.4197, 25.3572)
  line L7916 (-18.4197, 25.3572) -> (-18.4197, 26.3572)
  line L7917 (-18.4197, 26.3572) -> (-17.4197, 26.3572)
  line L7918 (-17.4197, 26.3572) -> (-17.4197, 25.3572)
  line L7919 (-17.9785, 25.3572) -> (-18.9785, 25.3572)
  line L7920 (-18.9785, 25.3572) -> (-18.9785, 26.3572)
  line L7921 (-18.9785, 26.3572) -> (-17.9785, 26.3572)
  line L7922 (-17.9785, 26.3572) -> (-17.9785, 25.3572)
  line L7923 (-18.6897, 25.3572) -> (-19.6897, 25.3572)
  line L7924 (-19.6897, 25.3572) -> (-19.6897, 26.3572)
  line L7925 (-19.6897, 26.3572) -> (-18.6897, 26.3572)
  line L7926 (-18.6897, 26.3572) -> (-18.6897, 25.3572)
  line L7927 (-19.2739, 25.3572) -> (-20.2739, 25.3572)
  line L7928 (-20.2739, 25.3572) -> (-20.2739, 26.3572)
  line L7929 (-20.2739, 26.3572) -> (-19.2739, 26.3572)
  line L7930 (-19.2739, 26.3572) -> (-19.2739, 25.3572)
  line L7931 (-19.693, 25.3572) -> (-20.693, 25.3572)
  line L7932 (-20.693, 25.3572) -> (-20.693, 26.3572)
  line L7933 (-20.693, 26.3572) -> (-19.693, 26.3572)
  line L7934 (-19.693, 26.3572) -> (-19.693, 25.3572)
  line L7935 (-20.0613, 25.3572) -> (-21.0613, 25.3572)
  line L7936 (-21.0613, 25.3572) -> (-21.0613, 26.3572)
  line L7937 (-21.0613, 26.3572) -> (-20.0613, 26.3572)
  line L7938 (-20.0613, 26.3572) -> (-20.0613, 25.3572)
  line L7939 (-20.4931, 25.3572) -> (-21.4931, 25.3572)
  line L7940 (-21.4931, 25.3572) -> (-21.4931, 26.3572)
  line L7941 (-21.4931, 26.3572) -> (-20.4931, 26.3572)
  line L7942 (-20.4931, 26.3572) -> (-20.4931, 25.3572)
  line L7943 (-21.217, 25.3572) -> (-22.217, 25.3572)
  line L7944 (-22.217, 25.3572) -> (-22.217, 26.3572)
  line L7945 (-22.217, 26.3572) -> (-21.217, 26.3572)
  line L7946 (-21.217, 26.3572) -> (-21.217, 25.3572)
  line L7947 (-21.8012, 25.3572) -> (-22.8012, 25.3572)
  line L7948 (-22.8012, 25.3572) -> (-22.8012, 26.3572)
  line L7949 (-22.8012, 26.3572) -> (-21.8012, 26.3572)
  line L7950 (-21.8012, 26.3572) -> (-21.8012, 25.3572)
  line L7951 (-12.962, 25.3826) -> (-13.962, 25.3826)
  line L7952 (-13.962, 25.3826) -> (-13.962, 26.3826)
  line L7953 (-13.962, 26.3826) -> (-12.962, 26.3826)
  line L7954 (-12.962, 26.3826) -> (-12.962, 25.3826)
  line L7955 (-14.6765, 25.3826) -> (-15.6765, 25.3826)
  line L7956 (-15.6765, 25.3826) -> (-15.6765, 26.3826)
  line L7957 (-15.6765, 26.3826) -> (-14.6765, 26.3826)
  line L7958 (-14.6765, 26.3826) -> (-14.6765, 25.3826)
  line L7959 (-15.5147, 25.3826) -> (-16.5147, 25.3826)
  line L7960 (-16.5147, 25.3826) -> (-16.5147, 26.3826)
  line L7961 (-16.5147, 26.3826) -> (-15.5147, 26.3826)
  line L7962 (-15.5147, 26.3826) -> (-15.5147, 25.3826)
  line L7963 (-16.2259, 25.3826) -> (-17.2259, 25.3826)
  line L7964 (-17.2259, 25.3826) -> (-17.2259, 26.3826)
  line L7965 (-17.2259, 26.3826) -> (-16.2259, 26.3826)
  line L7966 (-16.2259, 26.3826) -> (-16.2259, 25.3826)
  line L7967 (-16.7593, 25.3826) -> (-17.7593, 25.3826)
  line L7968 (-17.7593, 25.3826) -> (-17.7593, 26.3826)
  line L7969 (-17.7593, 26.3826) -> (-16.7593, 26.3826)
  line L7970 (-16.7593, 26.3826) -> (-16.7593, 25.3826)
  line L7971 (-17.4197, 25.3826) -> (-18.4197, 25.3826)
  line L7972 (-18.4197, 25.3826) -> (-18.4197, 26.3826)
  line L7973 (-18.4197, 26.3826) -> (-17.4197, 26.3826)
  line L7974 (-17.4197, 26.3826) -> (-17.4197, 25.3826)
  line L7975 (-17.9912, 25.3826) -> (-18.9912, 25.3826)
  line L7976 (-18.9912, 25.3826) -> (-18.9912, 26.3826)
  line L7977 (-18.9912, 26.3826) -> (-17.9912, 26.3826)
  line L7978 (-17.9912, 26.3826) -> (-17.9912, 25.3826)
  line L7979 (-18.6897, 25.3826) -> (-19.6897, 25.3826)
  line L7980 (-19.6897, 25.3826) -> (-19.6897, 26.3826)
  line L7981 (-19.6897, 26.3826) -> (-18.6897, 26.3826)
  line L7982 (-18.6897, 26.3826) -> (-18.6897, 25.3826)
  line L7983 (-19.2739, 25.3826) -> (-20.2739, 25.3826)
  line L7984 (-20.2739, 25.3826) -> (-20.2739, 26.3826)
  line L7985 (-20.2739, 26.3826) -> (-19.2739, 26.3826)
  line L7986 (-19.2739, 26.3826) -> (-19.2739, 25.3826)
  line L7987 (-19.693, 25.3826) -> (-20.693, 25.3826)
  line L7988 (-20.693, 25.3826) -> (-20.693, 26.3826)
  line L7989 (-20.693, 26.3826) -> (-19.693, 26.3826)
  line L7990 (-19.693, 26.3826) -> (-19.693, 25.3826)
  line L7991 (-20.0613, 25.3826) -> (-21.0613, 25.3826)
  line L7992 (-21.0613, 25.3826) -> (-21.0613, 26.3826)
  line L7993 (-21.0613, 26.3826) -> (-20.0613, 26.3826)
  line L7994 (-20.0613, 26.3826) -> (-20.0613, 25.3826)
  line L7995 (-20.4931, 25.3826) -> (-21.4931, 25.3826)
  line L7996 (-21.4931, 25.3826) -> (-21.4931, 26.3826)
  line L7997 (-21.4931, 26.3826) -> (-20.4931, 26.3826)
  line L7998 (-20.4931, 26.3826) -> (-20.4931, 25.3826)
  line L7999 (-21.217, 25.3826) -> (-22.217, 25.3826)
  line L8000 (-22.217, 25.3826) -> (-22.217, 26.3826)
  line L8001 (-22.217, 26.3826) -> (-21.217, 26.3826)
  line L8002 (-21.217, 26.3826) -> (-21.217, 25.3826)
  line L8003 (-21.8266, 25.3826) -> (-22.8266, 25.3826)
  line L8004 (-22.8266, 25.3826) -> (-22.8266, 26.3826)
  line L8005 (-22.8266, 26.3826) -> (-21.8266, 26.3826)
  line L8006 (-21.8266, 26.3826) -> (-21.8266, 25.3826)
  line L8007 (-12.9874, 25.408) -> (-13.9874, 25.408)
  line L8008 (-13.9874, 25.408) -> (-13.9874, 26.408)
  line L8009 (-13.9874, 26.408) -> (-12.9874, 26.408)
  line L8010 (-12.9874, 26.408) -> (-12.9874, 25.408)
  line L8011 (-14.7019, 25.408) -> (-15.7019, 25.408)
  line L8012 (-15.7019, 25.408) -> (-15.7019, 26.408)
  line L8013 (-15.7019, 26.408) -> (-14.7019, 26.408)
  line L8014 (-14.7019, 26.408) -> (-14.7019, 25.408)
  line L8015 (-15.5147, 25.408) -> (-16.5147, 25.408)
  line L8016 (-16.5147, 25.408) -> (-16.5147, 26.408)
  line L8017 (-16.5147, 26.408) -> (-15.5147, 26.408)
  line L8018 (-15.5147, 26.408) -> (-15.5147, 25.408)
  line L8019 (-16.2132, 25.408) -> (-17.2132, 25.408)
  line L8020 (-17.2132, 25.408) -> (-17.2132, 26.408)
  line L8021 (-17.2132, 26.408) -> (-16.2132, 26.408)
  line L8022 (-16.2132, 26.408) -> (-16.2132, 25.408)
  line L8023 (-16.7593, 25.408) -> (-17.7593, 25.408)
  line L8024 (-17.7593, 25.408) -> (-17.7593, 26.408)
  line L8025 (-17.7593, 26.408) -> (-16.7593, 26.408)
  line L8026 (-16.7593, 26.408) -> (-16.7593, 25.408)
  line L8027 (-17.4197, 25.408) -> (-18.4197, 25.408)
  line L8028 (-18.4197, 25.408) -> (-18.4197, 26.408)
  line L8029 (-18.4197, 26.408) -> (-17.4197, 26.408)
  line L8030 (-17.4197, 26.408) -> (-17.4197, 25.408)
  line L8031 (-18.0039, 25.408) -> (-19.0039, 25.408)
  line L8032 (-19.0039, 25.408) -> (-19.0039, 26.408)
  line L8033 (-19.0039, 26.408) -> (-18.0039, 26.408)
  line L8034 (-18.0039, 26.408) -> (-18.0039, 25.408)
  line L8035 (-18.677, 25.408) -> (-19.677, 25.408)
  line L8036 (-19.677, 25.408) -> (-19.677, 26.408)
  line L8037 (-19.677, 26.408) -> (-18.677, 26.408)
  line L8038 (-18.677, 26.408) -> (-18.677, 25.408)
  line L8039 (-19.2739, 25.408) -> (-20.2739, 25.408)
  line L8040 (-20.2739, 25.408) -> (-20.2739, 26.408)
  line L8041 (-20.2739, 26.408) -> (-19.2739, 26.408)
  line L8042 (-19.2739, 26.408) -> (-19.2739, 25.408)
  line L8043 (-19.693, 25.408) -> (-20.693, 25.408)
  line L8044 (-20.693, 25.408) -> (-20.693, 26.408)
  line L8045 (-20.693, 26.408) -> (-19.693, 26.408)
  line L8046 (-19.693, 26.408) -> (-19.693, 25.408)
  line L8047 (-20.0867, 25.408) -> (-21.0867, 25.408)
  line L8048 (-21.0867, 25.408) -> (-21.0867, 26.408)
  line L8049 (-21.0867, 26.408) -> (-20.0867, 26.408)
  line L8050 (-20.0867, 26.408) -> (-20.0867, 25.408)
  line L8051 (-20.4931, 25.408) -> (-21.4931, 25.408)
  line L8052 (-21.4931, 25.408) -> (-21.4931, 26.408)
  line L8053 (-21.4931, 26.408) -> (-20.4931, 26.408)
  line L8054 (-20.4931, 26.408) -> (-20.4931, 25.408)
  line L8055 (-21.2043, 25.408) -> (-22.2043, 25.408)
  line L8056 (-22.2043, 25.408) -> (-22.2043, 26.408)
  line L8057 (-22.2043, 26.408) -> (-21.2043, 26.408)
  line L8058 (-21.2043, 26.408) -> (-21.2043, 25.408)
  line L8059 (-21.8266, 25.408) -> (-22.8266, 25.408)
  line L8060 (-22.8266, 25.408) -> (-22.8266, 26.408)
  line L8061 (-22.8266, 26.408) -> (-21.8266, 26.408)
  line L8062 (-21.8266, 26.408) -> (-21.8266, 25.408)
  line L8063 (-13.0128, 25.4334) -> (-14.0128, 25.4334)
  line L8064 (-14.0128, 25.4334) -> (-14.0128, 26.4334)
  line L8065 (-14.0128, 26.4334) -> (-13.0128, 26.4334)
  line L8066 (-13.0128, 26.4334) -> (-13.0128, 25.4334)
  line L8067 (-14.7273, 25.4334) -> (-15.7273, 25.4334)
  line L8068 (-15.7273, 25.4334) -> (-15.7273, 26.4334)
  line L8069 (-15.7273, 26.4334) -> (-14.7273, 26.4334)
  line L8070 (-14.7273, 26.4334) -> (-14.7273, 25.4334)
  line L8071 (-15.5147, 25.4334) -> (-16.5147, 25.4334)
  line L8072 (-16.5147, 25.4334) -> (-16.5147, 26.4334)
  line L8073 (-16.5147, 26.4334) -> (-15.5147, 26.4334)
  line L8074 (-15.5147, 26.4334) -> (-15.5147, 25.4334)
  line L8075 (-16.2005, 25.4334) -> (-17.2005, 25.4334)
  line L8076 (-17.2005, 25.4334) -> (-17.2005, 26.4334)